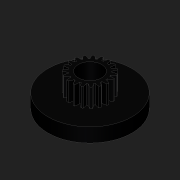
# Autodesk Inventor part: SE01
Saved by Autodesk Inventor 2017 (Build 210142000, 142)
## iProperties
Created: 2019-09-07
Part Number: SE01
Material: ABS Plastic
Document SubType Name: Modeling
Designer: Dell
Density: 1.06 g/cm^3
Appearance: Smooth - Black
Author: Dell
Autodesk Inventor part; units mm, degrees
ref_plane "YZ Plane" through (0, 0, 0) normal (1, 0, 0) x (0, 1, 0)
ref_plane "XZ Plane" through (0, 0, 0) normal (0, 1, 0) x (-1, 0, 0)
ref_plane "XY Plane" through (0, 0, 0) normal (0, 0, 1) x (1, 0, 0)
sketch "Sketch1" plane through (0, 0, 0) normal (0, 0, 1) x (1, 0, 0)
  circle A0 centre (0, 0) radius 45
  dimension "d0" = 90
  constraints: 1 centre point, 1 coincident
  measures "d0" diameter of A0
extrude "Extrusion1" add sketch "Sketch1" along normal blind 5
sketch "Sketch2" plane through (0, 0, 5) normal (0, 0, 1) x (1, 0, 0)
  circle A0 centre (0, 0) radius 15
  dimension "d3" = 30
  constraints: 1 centre point, 1 coincident
  measures "d3" diameter of A0
extrude "Extrusion2" add sketch "Sketch2" along normal blind 20
sketch "Sketch3" plane through (0, 0, 0) normal (0, 0, -1) x (-1, 0, 0)
  circle A0 centre (0, 0) radius 45 projected
  circle A1 centre (0, 0) radius 40
  dimension "d6" = 80
  constraints: 1 centre point, 1 coincident
  measures "d6" diameter of A1
extrude "Extrusion3" add sketch "Sketch3" along normal blind 10
sketch "Sketch8" plane through (0, 0, 25) normal (0, 0, 1) x (1, 0, 0)
  circle A0 centre (0, 0) radius 12.5
  dimension "d35" = 25
  constraints: 1 centre point, 1 coincident
  measures "d35" diameter of A0
extrude "Extrusion7" cut sketch "Sketch8" against normal through all
sketch "Sketch9" plane through (0, 0, 0) normal (0, 0, -1) x (-1, 0, 0)
  circle A0 centre (0, 0) radius 18.415 construction
  circle A1 centre (0, 0) radius 4.7625 construction
  circle A2 centre (0, 0) radius 15.494 construction
  line L0 (0, 18.415) -> (-38.1, 18.415) construction
  line L1 (-38.1, 18.415) -> (-38.1, 15.494) construction
  line L2 (-38.1, 15.494) -> (0, 15.494) construction
  line L3 (0, 18.415) -> (0, 15.494) construction
  circle A3 centre (0, 0) radius 45 construction
  line L4 (0, 45) -> (0, 19.415)
  circle A4 centre (0, 0) radius 19.415 construction
  line L5 (0, 19.415) -> (-40.5963, 19.415)
  arc A5 (0, 45) -> (-40.5963, 19.415) centre (0, 0) ccw
  line L6 (-12.9177, 14.494) -> (-42.6019, 14.494)
  arc A6 (-12.9177, 14.494) -> (-19.415, 0) centre (0, 0) ccw
  line L7 (-19.415, 0) -> (-45, 0)
  arc A7 (-42.6019, 14.494) -> (-45, 0) centre (0, 0) ccw
  arc A8 (-40.5963, 19.415) -> (-42.6019, 14.494) centre (0, 0) ccw
  line L8 (-39.1, 19.415) -> (-39.1, 14.494)
  circle A9 centre (0, 0) radius 45 projected
  arc A10 (0, 19.415) -> (-12.9177, 14.494) centre (0, 0) ccw
  dimension "d38" = 36.83
  dimension "d39" = 30.988
  dimension "d40" = 38.1
  dimension "d41" = 1
  dimension "d42" = 1
  dimension "d43" = 1
  dimension "d44" = 1
  constraints: 18 end point, 17 point on circle, 8 centre point, 6 coincident, 6 horizontal, 4 concentric, 3 perpendicular, 3 vertical alignment, 2 horizontal alignment, 2 point on line, 1 vertical, 5 other
  measures "d40" distance of L0.start L0.end
  measures "d42" distance between parallel lines of L5 L0
  measures "d43" distance between parallel lines of L6 L2
  measures "d44" distance between parallel lines of L1 L8
extrude "Extrusion8" add sketch "Sketch9" along normal blind 10 contours L4 L5 A5 | A6 L7 A7 L6
extrude "Extrusion9" cut sketch "Sketch9" along normal through all contours A10 L6 L8 L5 | L5 L8 L6 A8
sketch "Sketch17" plane through (0, 0, 0) normal (0, 0, -1) x (-1, 0, 0)
  line L0 (-40, 0) -> (-19.415, 0) projected
  circle A0 centre (0, 0) radius 40
  line L1 (-12.9177, 14.494) -> (-42.6019, 14.494) projected
  circle A1 centre (0, 0) radius 45
  line L2 (-40.5963, 19.415) -> (0, 19.415) projected
  arc A2 (-40.5963, 19.415) -> (-42.6019, 14.494) centre (0, 0) ccw
  arc A3 (-34.9722, 19.415) -> (-37.2817, 14.494) centre (0, 0) ccw
  line L3 (-42.6019, 14.494) -> (-37.2817, 14.494)
  line L4 (-34.9722, 19.415) -> (-40.5963, 19.415)
  constraints: 7 point on circle, 4 end point, 3 centre point, 2 coincident, 2 point on line, 1 collinear, 1 concentric, 1 parallel, 4 other
extrude "Extrusion17" add sketch "Sketch17" along normal blind 10 contours A0 L1 A1 L2 picked at (-37.6663, 17.7979)
sketch "Sketch18" plane through (0, 0, 5) normal (0, 0, 1) x (1, 0, 0)
  circle A0 centre (0, 0) radius 12.5
  arc A1 (-7.6337, 19.5634) -> (-7.2467, 14.8235) centre (8.4724, 18.4924) ccw
  arc A2 (-7.2467, 14.8235) -> (-8.4461, 14.1744) centre (0, 0) ccw
  arc A3 (-8.4461, 14.1744) -> (-12.2026, 17.0908) centre (-20.1151, 3.0216) ccw
  arc A4 (-12.2026, 17.0908) -> (-13.5723, 16.0248) centre (0, 0) ccw
  arc A5 (-13.5723, 16.0248) -> (-11.6673, 11.6673) centre (2.0089, 20.2414) ccw
  arc A6 (-11.6673, 11.6673) -> (-12.5909, 10.6639) centre (0, 0) ccw
  arc A7 (-12.5909, 10.6639) -> (-17.0908, 12.2026) centre (-20.0064, -3.6735) ccw
  arc A8 (-17.0908, 12.2026) -> (-18.0401, 10.7496) centre (0, 0) ccw
  arc A9 (-18.0401, 10.7496) -> (-14.8235, 7.2467) centre (-4.6724, 19.7969) ccw
  arc A10 (-14.8235, 7.2467) -> (-15.3713, 5.9979) centre (0, 0) ccw
  arc A11 (-15.3713, 5.9979) -> (-20.127, 5.9921) centre (-17.7296, -9.9705) ccw
  arc A12 (-20.127, 5.9921) -> (-20.5531, 4.3095) centre (0, 0) ccw
  arc A13 (-20.5531, 4.3095) -> (-16.3733, 2.0409) centre (-10.8472, 17.2072) ccw
  arc A14 (-16.3733, 2.0409) -> (-16.4859, 0.6819) centre (0, 0) ccw
  arc A15 (-16.4859, 0.6819) -> (-20.9821, -0.8678) centre (-13.5315, -15.1871) ccw
  arc A16 (-20.9821, -0.8678) -> (-20.8387, -2.5975) centre (0, 0) ccw
  arc A17 (-20.8387, -2.5975) -> (-16.1488, -3.3861) centre (-15.8467, 12.7527) ccw
  arc A18 (-16.1488, -3.3861) -> (-15.8141, -4.708) centre (0, 0) ccw
  arc A19 (-15.8141, -4.708) -> (-19.5634, -7.6337) centre (-7.8671, -18.7579) ccw
  arc A20 (-19.5634, -7.6337) -> (-18.8662, -9.2231) centre (0, 0) ccw
  arc A21 (-18.8662, -9.2231) -> (-14.1744, -8.4461) centre (-19.1289, 6.9163) ccw
  arc A22 (-14.1744, -8.4461) -> (-13.4285, -9.5878) centre (0, 0) ccw
  arc A23 (-13.4285, -9.5878) -> (-16.0248, -13.5723) centre (-1.3502, -20.296) ccw
  arc A24 (-16.0248, -13.5723) -> (-14.8492, -14.8492) centre (0, 0) ccw
  arc A25 (-14.8492, -14.8492) -> (-10.6639, -12.5909) centre (-20.3381, 0.3305) ccw
  arc A26 (-10.6639, -12.5909) -> (-9.5878, -13.4285) centre (0, 0) ccw
  arc A27 (-9.5878, -13.4285) -> (-10.7496, -18.0401) centre (5.3131, -19.6347) ccw
  arc A28 (-10.7496, -18.0401) -> (-9.2231, -18.8662) centre (0, 0) ccw
  arc A29 (-9.2231, -18.8662) -> (-5.9979, -15.3713) centre (-19.3435, -6.2912) ccw
  arc A30 (-5.9979, -15.3713) -> (-4.708, -15.8141) centre (0, 0) ccw
  arc A31 (-4.708, -15.8141) -> (-4.3095, -20.5531) centre (11.4006, -16.8457) ccw
  arc A32 (-4.3095, -20.5531) -> (-2.5975, -20.8387) centre (0, 0) ccw
  arc A33 (-2.5975, -20.8387) -> (-0.6819, -16.4859) centre (-16.2526, -12.2312) ccw
  arc A34 (-0.6819, -16.4859) -> (0.6819, -16.4859) centre (0, 0) ccw
  arc A35 (0.6819, -16.4859) -> (2.5975, -20.8387) centre (16.2526, -12.2312) ccw
  arc A36 (2.5975, -20.8387) -> (4.3095, -20.5531) centre (0, 0) ccw
  arc A37 (4.3095, -20.5531) -> (4.708, -15.8141) centre (-11.4006, -16.8457) ccw
  arc A38 (4.708, -15.8141) -> (5.9979, -15.3713) centre (0, 0) ccw
  arc A39 (5.9979, -15.3713) -> (9.2231, -18.8662) centre (19.3435, -6.2912) ccw
  arc A40 (9.2231, -18.8662) -> (10.7496, -18.0401) centre (0, 0) ccw
  arc A41 (10.7496, -18.0401) -> (9.5878, -13.4285) centre (-5.3131, -19.6347) ccw
  arc A42 (9.5878, -13.4285) -> (10.6639, -12.5909) centre (0, 0) ccw
  arc A43 (10.6639, -12.5909) -> (14.8492, -14.8492) centre (20.3381, 0.3305) ccw
  arc A44 (14.8492, -14.8492) -> (16.0248, -13.5723) centre (0, 0) ccw
  arc A45 (16.0248, -13.5723) -> (13.4285, -9.5878) centre (1.3502, -20.296) ccw
  arc A46 (13.4285, -9.5878) -> (14.1744, -8.4461) centre (0, 0) ccw
  arc A47 (14.1744, -8.4461) -> (18.8662, -9.2231) centre (19.1289, 6.9163) ccw
  arc A48 (18.8662, -9.2231) -> (19.5634, -7.6337) centre (0, 0) ccw
  arc A49 (19.5634, -7.6337) -> (15.8141, -4.708) centre (7.8671, -18.7579) ccw
  arc A50 (15.8141, -4.708) -> (16.1488, -3.3861) centre (0, 0) ccw
  arc A51 (16.1488, -3.3861) -> (20.8387, -2.5975) centre (15.8467, 12.7527) ccw
  arc A52 (20.8387, -2.5975) -> (20.9821, -0.8678) centre (0, 0) ccw
  arc A53 (20.9821, -0.8678) -> (16.4859, 0.6819) centre (13.5315, -15.1871) ccw
  arc A54 (16.4859, 0.6819) -> (16.3733, 2.0409) centre (0, 0) ccw
  arc A55 (16.3733, 2.0409) -> (20.5531, 4.3095) centre (10.8472, 17.2072) ccw
  arc A56 (20.5531, 4.3095) -> (20.127, 5.9921) centre (0, 0) ccw
  arc A57 (20.127, 5.9921) -> (15.3713, 5.9979) centre (17.7296, -9.9705) ccw
  arc A58 (15.3713, 5.9979) -> (14.8235, 7.2467) centre (0, 0) ccw
  arc A59 (14.8235, 7.2467) -> (18.0401, 10.7496) centre (4.6724, 19.7969) ccw
  arc A60 (18.0401, 10.7496) -> (17.0908, 12.2026) centre (0, 0) ccw
  arc A61 (17.0908, 12.2026) -> (12.5909, 10.6639) centre (20.0064, -3.6735) ccw
  arc A62 (12.5909, 10.6639) -> (11.6673, 11.6673) centre (0, 0) ccw
  arc A63 (11.6673, 11.6673) -> (13.5723, 16.0248) centre (-2.0089, 20.2414) ccw
  arc A64 (13.5723, 16.0248) -> (12.2026, 17.0908) centre (0, 0) ccw
  arc A65 (12.2026, 17.0908) -> (8.4461, 14.1744) centre (20.1151, 3.0216) ccw
  arc A66 (8.4461, 14.1744) -> (7.2467, 14.8235) centre (0, 0) ccw
  arc A67 (7.2467, 14.8235) -> (7.6337, 19.5634) centre (-8.4724, 18.4924) ccw
  arc A68 (7.6337, 19.5634) -> (5.9921, 20.127) centre (0, 0) ccw
  arc A69 (5.9921, 20.127) -> (3.3861, 16.1488) centre (18.0441, 9.3892) ccw
  arc A70 (3.3861, 16.1488) -> (2.0409, 16.3733) centre (0, 0) ccw
  arc A71 (2.0409, 16.3733) -> (0.8678, 20.9821) centre (-14.0178, 14.7394) ccw
  arc A72 (0.8678, 20.9821) -> (-0.8678, 20.9821) centre (0, 0) ccw
  arc A73 (-0.8678, 20.9821) -> (-2.0409, 16.3733) centre (14.0178, 14.7394) ccw
  arc A74 (-2.0409, 16.3733) -> (-3.3861, 16.1488) centre (0, 0) ccw
  arc A75 (-3.3861, 16.1488) -> (-5.9921, 20.127) centre (-18.0441, 9.3892) ccw
  arc A76 (-5.9921, 20.127) -> (-7.6337, 19.5634) centre (0, 0) ccw
  constraints: 152 point on circle, 77 centre point
extrude "Extrusion18" add sketch "Sketch18" along normal blind 20
body "Solid1"
